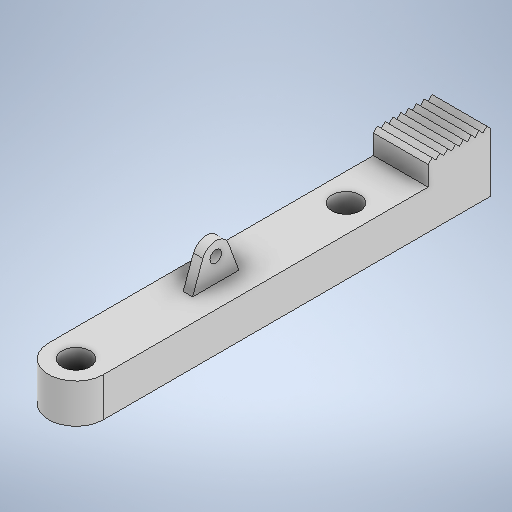
# Autodesk Inventor part: Gripper_arms
Saved by Autodesk Inventor 2025.2 (Build 292293000, 293)
## iProperties
Created: 2025-01-12
Part Number: Gripper_arms
Material: Generic
Document SubType Name: Modeling
Designer: caomi
Density: 1 g/cm^3
Appearance: Default
Author: caomi
Autodesk Inventor part; units mm, degrees
ref_plane "YZ Plane" through (0, 0, 0) normal (1, 0, 0) x (0, 1, 0)
ref_plane "XZ Plane" through (0, 0, 0) normal (0, 1, 0) x (-1, 0, 0)
ref_plane "XY Plane" through (0, 0, 0) normal (0, 0, 1) x (1, 0, 0)
sketch "Sketch1" plane through (0, 0, 0) normal (0, 1, 0) x (-1, 0, 0)
  line L0 (-7, 41.5) -> (7, 41.5)
  line L1 (7, 41.5) -> (7, -41.5)
  line L2 (7, -41.5) -> (-7, -41.5)
  line L3 (-7, -41.5) -> (-7, 41.5)
  line L4 (-7, 41.5) -> (7, -41.5) construction
  line L5 (7, 41.5) -> (-7, -41.5) construction
  circle A0 centre (0, 34.5) radius 3.6
  circle A1 centre (0, -34.5) radius 3.6
  line L6 (13.7936, 0) -> (-15.5073, 0) construction
  point P0 (0, 0)
  dimension "d0" = 7.2
  dimension "d1" = 69
  dimension "d2" = 83
  dimension "d3" = 14
  constraints: 14 end point, 2 centre point, 2 horizontal, 2 midpoint, 2 parallel, 2 vertical alignment, 1 perpendicular, 1 point on line, 1 other
  measures "d0" diameter of A0
  measures "d1" distance of A0.centre A1.centre
  measures "d2" distance of L0.end L1.end
  measures "d3" distance of L0.start L0.end
extrude "Extrusion1" add sketch "Sketch1" along normal mid plane 10
sketch "Sketch2" plane through (0, 0, 0) normal (1, 0, 0) x (0, 1, 0)
  circle A0 centre (11, 0) radius 3.5
  line L0 (12.1971, -3.2889) -> (5, -5.9084)
  line L1 (5, -41.5) -> (5, 41.5) projected
  line L2 (12.1971, 3.2889) -> (5, 5.9084)
  line L3 (11, 0) -> (-7.9221, 0) construction
  circle A1 centre (11, 0) radius 1.5
  point P0 (0, 0)
  point P1 (16.3025, 1.2439)
  point P2 (5, 7.6173)
  point P3 (5, -5.09)
  point P4 (5, 0)
  dimension "d6" = 7
  dimension "d11" = 20
  dimension "d12" = 6
  dimension "d13" = 3
  constraints: 6 end point, 2 centre point, 2 point on circle, 2 point on line, 1 horizontal, 1 horizontal alignment, 1 midpoint, 1 tangent, 1 other
  measures "d6" diameter of A0
  measures "d11" angle of L3 L2
  measures "d12" distance of point (5, 0) L3.start
  measures "d13" diameter of A1
extrude "Extrusion2" add sketch "Sketch2" along normal mid plane 2.4
fillet "Fillet1" radius 7 4 edges at (-7, 0, 41.5) (7, 0, 41.5) (-7, 0, -41.5) (7, 0, -41.5)
sketch "Sketch3" plane through (0, 5, 0) normal (0, 1, 0) x (1, 0, 0)
  line L0 (-7, 34.5) -> (-7, 64.5)
  line L1 (-7, 64.5) -> (7, 64.5)
  line L2 (7, 64.5) -> (7, 34.5)
  circle A0 centre (0, 34.5) radius 3.6 projected
  point P0 (0, 0)
  dimension "d30" = 30
  constraints: 6 end point, 2 coincident, 1 horizontal, 1 parallel, 1 vertical
  measures "d30" distance from line of A0.centre L1
extrude "Extrusion3" add sketch "Sketch3" against normal up to surface (10 mm away) fills toward (-6.95, 49.5) open curves L0 L1 L2
sketch "Sketch4" plane through (-7, -5, -34.5) normal (-1, 0, 0) x (0, 0, 1)
  line L0 (-14, 10) -> (-30, 10)
  line L1 (-30, 10) -> (-30, 15)
  line L2 (-30, 15) -> (-14, 15)
  line L3 (-14, 15) -> (-14, 10)
  line L4 (-30, 15) -> (-29, 16)
  line L5 (-29, 16) -> (-28, 15)
  line L6 (-29, 16) -> (-29, 13.5033) construction
  line L7 (-28, 15) -> (-27, 16)
  line L8 (-27, 16) -> (-26, 15)
  line L9 (-26, 15) -> (-25, 16)
  line L10 (-25, 16) -> (-24, 15)
  line L11 (-24, 15) -> (-23, 16)
  line L12 (-23, 16) -> (-22, 15)
  line L13 (-22, 15) -> (-21, 16)
  line L14 (-21, 16) -> (-20, 15)
  line L15 (-20, 15) -> (-19, 16)
  line L16 (-19, 16) -> (-18, 15)
  line L17 (-18, 15) -> (-17, 16)
  line L18 (-17, 16) -> (-16, 15)
  line L19 (-16, 15) -> (-15, 16)
  line L20 (-15, 16) -> (-14, 15)
  point P0 (-14, 15)
  point P1 (-16, 15)
  point P2 (-18, 15)
  point P3 (-20, 15)
  point P4 (-22, 15)
  point P5 (-24, 15)
  point P6 (-26, 15)
  point P7 (-28, 15)
  point P8 (-14, 15)
  point P9 (-16, 15)
  point P10 (-16, 15)
  point P11 (-18, 15)
  point P12 (-18, 15)
  point P13 (-20, 15)
  point P14 (-20, 15)
  point P15 (-22, 15)
  point P16 (-22, 15)
  dimension "d17" = 45
  dimension "d18" = 1
  dimension "d21" = 2
  dimension "d26" = 16
  dimension "d27" = 5
  constraints: 42 end point, 2 horizontal, 2 parallel, 1 perpendicular, 1 point on line, 1 vertical, 36 other
  measures "d17" angle of L2 L4
  measures "d18" distance from line of L2 L4.end
  measures "d21" distance of L1.end L7.start
  measures "d26" distance between parallel lines of L3 L1
  measures "d27" distance between parallel lines of L0 L2
extrude "Extrusion4" add sketch "Sketch4" against normal up to surface (14 mm away)
equation "\"d10\" = 0.5 * d3"
body "Solid1"
